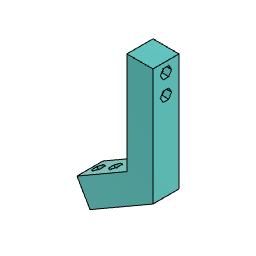
upper_middle_frame (Autodesk Fusion 360 design; units mm, degrees)
Autodesk Fusion 360 part; units mm, degrees
sketch "Sketch1" plane through (0, 0, 0) normal (0, 1, 0) x (1, 0, 0)
  line L0 (0, 0) -> (26.1117, 0) construction
  line L1 (0, 0) -> (43.3013, -25)
  line L2 (43.3013, -25) -> (43.3013, -109)
  dimension "d1" = 50
  dimension "d2" = 30
  dimension "d3" = 84
  constraint coincident L0.start L1.start
  constraint horizontal L0
  constraint perpendicular L0 L2
  measures "d1" distance of L0.start L1.end
  measures "d2" angle of L0 L1
  measures "d3" distance of L1.end L2.end
pipe "Pipe1" add square section size 20 path "Sketch1" along L1 L2
sketch "Sketch2" plane through (-5, 0, 8.6603) normal (-0.5, 0, 0.866025) x (0, -1, 0)
  line L0 (-10, 0) -> (10, 0)
  line L1 (10, 0) -> (10, 44.2265)
  line L2 (10, 44.2265) -> (-10, 44.2265)
  line L3 (-10, 44.2265) -> (-10, 0)
  line L4 (0, 0) -> (0, 44.2265) construction
  circle A0 centre (0, 7.5) radius 2
  circle A1 centre (0, 22.5) radius 2
  line L5 (2.1362, 3.8) -> (4.2724, 7.5)
  line L6 (4.2724, 7.5) -> (2.1362, 11.2)
  line L7 (2.1362, 11.2) -> (-2.1362, 11.2)
  line L8 (-2.1362, 11.2) -> (-4.2724, 7.5)
  line L9 (-4.2724, 7.5) -> (-2.1362, 3.8)
  line L10 (-2.1362, 3.8) -> (2.1362, 3.8)
  line L11 (2.1362, 18.8) -> (4.2724, 22.5)
  line L12 (4.2724, 22.5) -> (2.1362, 26.2)
  line L13 (2.1362, 26.2) -> (-2.1362, 26.2)
  line L14 (-2.1362, 26.2) -> (-4.2724, 22.5)
  line L15 (-4.2724, 22.5) -> (-2.1362, 18.8)
  line L16 (-2.1362, 18.8) -> (2.1362, 18.8)
  point P0 (0, 7.5)
  point P1 (0, 22.5)
  dimension "d8" = 4
  dimension "d9" = 7.5
  dimension "d10" = 15
  dimension "d11" = 7.4
  constraint coincident L4.start origin
  constraint midpoint L2 L4.end
  constraint coincident L4 P0
  constraint coincident L4 P1
  constraint equal A0 A1
  constraint coincident P0 A0.centre
  constraint coincident P1 A1.centre
  constraint vertical L5.end L11.end
  constraint horizontal L10
  constraint horizontal L16
  measures "d8" diameter of A1
  measures "d9" distance of L4.start A0.centre
  measures "d10" distance of P0 P1
  measures "d11" distance of L7 L10
extrude "Extrude1" cut sketch "Sketch2" against normal blind 40 contours A0 | A1
extrude "Extrude2" cut sketch "Sketch2" against normal blind 5 contours L5 L6 L7 L8 L9 L10 | L11 L12 L13 L14 L15 L16
sketch "Sketch3" plane through (53.3013, 0, 0) normal (1, 0, 0) x (0, 1, 0)
  line L0 (-10, 19.2265) -> (10, 19.2265)
  line L1 (10, 19.2265) -> (10, 109)
  line L2 (10, 109) -> (-10, 109)
  line L3 (-10, 109) -> (-10, 19.2265)
  line L4 (0, 109) -> (0, 74.4412) construction
  circle A0 centre (0, 101.5) radius 2
  circle A1 centre (0, 86.5) radius 2
  line L5 (-2.1362, 105.2) -> (-4.2724, 101.5)
  line L6 (-4.2724, 101.5) -> (-2.1362, 97.8)
  line L7 (-2.1362, 97.8) -> (2.1362, 97.8)
  line L8 (2.1362, 97.8) -> (4.2724, 101.5)
  line L9 (4.2724, 101.5) -> (2.1362, 105.2)
  line L10 (2.1362, 105.2) -> (-2.1362, 105.2)
  line L11 (-2.1362, 90.2) -> (-4.2724, 86.5)
  line L12 (-4.2724, 86.5) -> (-2.1362, 82.8)
  line L13 (-2.1362, 82.8) -> (2.1362, 82.8)
  line L14 (2.1362, 82.8) -> (4.2724, 86.5)
  line L15 (4.2724, 86.5) -> (2.1362, 90.2)
  line L16 (2.1362, 90.2) -> (-2.1362, 90.2)
  point P0 (0, 101.5)
  point P1 (0, 86.5)
  dimension "d17" = 4
  dimension "d18" = 7.5
  dimension "d19" = 15
  dimension "d20" = 7.4
  constraint midpoint L2 L4.start
  constraint perpendicular L2 L4
  constraint coincident L4 P0
  constraint coincident L4 P1
  constraint equal A0 A1
  constraint coincident P0 A0.centre
  constraint coincident P1 A1.centre
  constraint equal L10 L16
  constraint horizontal L10
  constraint horizontal L16
  measures "d17" diameter of A0
  measures "d18" distance of L4.start P0
  measures "d19" distance of P0 P1
  measures "d20" distance of L7 L10
extrude "Extrude3" cut sketch "Sketch3" against normal blind 55 contours A0 | A1
extrude "Extrude4" cut sketch "Sketch3" against normal blind 5 contours L5 L6 L7 L8 L9 L10 | L11 L12 L13 L14 L15 L16
equation "d11 = 7 mm + 2 * gap"
equation "gap = 0.2 mm"
equation "d20 = 7 mm + 2 * gap"
